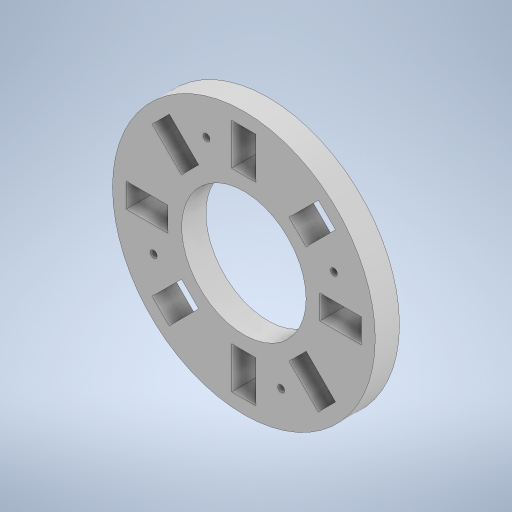
# Autodesk Inventor part: Spodnji obroc
Saved by Autodesk Inventor 2023 (Build 270158000, 158)
## iProperties
Created: 2022-12-16
Part Number: Spodnji obroc
Material: Generic
Document SubType Name: Modeling
Designer: David Zindović
Density: 1 g/cm^3
Appearance: Default
Author: David Zindović
Autodesk Inventor part; units mm, degrees
ref_plane "YZ Plane" through (0, 0, 0) normal (1, 0, 0) x (0, 1, 0)
ref_plane "XZ Plane" through (0, 0, 0) normal (0, 1, 0) x (-1, 0, 0)
ref_plane "XY Plane" through (0, 0, 0) normal (0, 0, 1) x (1, 0, 0)
sketch "Sketch1" plane through (0, 0, 0) normal (0, 0, 1) x (1, 0, 0)
  circle A0 centre (0, 0) radius 11
  circle A1 centre (0, 0) radius 17
  line L0 (11, 1.75) -> (17, 1.75)
  line L1 (17, 1.75) -> (17, -1.75)
  line L2 (17, -1.75) -> (11, -1.75)
  line L3 (11, -1.75) -> (11, 1.75)
  line L4 (13.2583, 10.7834) -> (9.0156, 6.5407)
  line L5 (9.0156, 6.5407) -> (6.5407, 9.0156)
  line L6 (6.5407, 9.0156) -> (10.7834, 13.2583)
  line L7 (10.7834, 13.2583) -> (13.2583, 10.7834)
  line L8 (1.75, 17) -> (1.75, 11)
  line L9 (1.75, 11) -> (-1.75, 11)
  line L10 (-1.75, 11) -> (-1.75, 17)
  line L11 (-1.75, 17) -> (1.75, 17)
  line L12 (-10.7834, 13.2583) -> (-6.5407, 9.0156)
  line L13 (-6.5407, 9.0156) -> (-9.0156, 6.5407)
  line L14 (-9.0156, 6.5407) -> (-13.2583, 10.7834)
  line L15 (-13.2583, 10.7834) -> (-10.7834, 13.2583)
  line L16 (-17, 1.75) -> (-11, 1.75)
  line L17 (-11, 1.75) -> (-11, -1.75)
  line L18 (-11, -1.75) -> (-17, -1.75)
  line L19 (-17, -1.75) -> (-17, 1.75)
  line L20 (-13.2583, -10.7834) -> (-9.0156, -6.5407)
  line L21 (-9.0156, -6.5407) -> (-6.5407, -9.0156)
  line L22 (-6.5407, -9.0156) -> (-10.7834, -13.2583)
  line L23 (-10.7834, -13.2583) -> (-13.2583, -10.7834)
  line L24 (-1.75, -17) -> (-1.75, -11)
  line L25 (-1.75, -11) -> (1.75, -11)
  line L26 (1.75, -11) -> (1.75, -17)
  line L27 (1.75, -17) -> (-1.75, -17)
  line L28 (10.7834, -13.2583) -> (6.5407, -9.0156)
  line L29 (6.5407, -9.0156) -> (9.0156, -6.5407)
  line L30 (9.0156, -6.5407) -> (13.2583, -10.7834)
  line L31 (13.2583, -10.7834) -> (10.7834, -13.2583)
  circle A2 centre (0, 0) radius 9
  circle A3 centre (0, 0) radius 19
  line L32 (-13.035, -5.3993) -> (-5.3993, 13.035)
  line L33 (-5.3993, 13.035) -> (13.035, 5.3993)
  line L34 (13.035, 5.3993) -> (5.3993, -13.035)
  line L35 (5.3993, -13.035) -> (-13.035, -5.3993)
  line L36 (0, 0) -> (-5.3993, 13.035)
  line L37 (0, 0) -> (14.109, 0) construction
  line L38 (0, 0) -> (16.0476, 6.6471)
  line L39 (0, 0) -> (17.3698, 0) construction
  circle A4 centre (-5.3993, 13.035) radius 0.5
  circle A5 centre (13.035, 5.3993) radius 0.5
  circle A6 centre (5.3993, -13.035) radius 0.5
  circle A7 centre (-13.035, -5.3993) radius 0.5
  point P0 (11, 0)
  point P1 (7.7782, 7.7782)
  point P2 (0, 11)
  point P3 (-7.7782, 7.7782)
  point P4 (-11, 0)
  point P5 (-7.7782, -7.7782)
  point P6 (0, -11)
  point P7 (7.7782, -7.7782)
  dimension "d0" = 22
  dimension "d1" = 6
  dimension "d2" = 3.5
  dimension "d3" = 6
  dimension "d6" = 360
  dimension "d8" = 2
  dimension "d9" = 2
  dimension "d23" = 112.5
  dimension "d24" = 22.5
  dimension "d25" = 1
  dimension "d26" = 1
  dimension "d27" = 1
  dimension "d28" = 1
  dimension "d29" = 14.109
  dimension "d30" = 19.9531
  dimension "d31" = 19.9531
  constraints: 81 end point, 8 centre point, 4 parallel, 3 coincident, 3 horizontal, 2 equal length, 2 perpendicular, 1 horizontal alignment, 1 midpoint, 1 point on line, 73 other
  measures "d0" diameter of A0
  measures "d1" radial gap between concentric circles of A0 A1
  measures "d2" distance of L2.end L0.start
  measures "d3" distance of L0.start L0.end
  measures "d8" radial gap between concentric circles of A0 A2
  measures "d9" radial gap between concentric circles of A1 A3
  measures "d23" angle of L37 L36
  measures "d24" angle of L39 L38
  measures "d25" diameter of A4
  measures "d26" diameter of A5
  measures "d27" diameter of A6
  measures "d28" diameter of A7
  measures "d29" distance of L36.start L32.end
  measures "d30" distance of L32.end L33.end
  measures "d31" distance of L33.end L34.end
extrude "Extrusion1" add sketch "Sketch1" along normal mid plane 3.5 contours A0 L34 | L3 L2 A1 L30 L29 A0 | A0 L34 L3 | L34 A0 L35 L32 L36 A2 L38 | A0 L38 A5 L34 L0 L3 | L29 L34 A0 | L38 A2 L36 A0 L33 | A0 L33 L5 L4 A5 L38 | L34 L29 L28 A6 L35 L26 L25 A0 | L34 A5 L38 A1 L0 | L33 A0 | A0 L5 L33 | L35 L25 A0 | A0 L35 | L28 A1 L26 L35 A6 L34 | A0 L9 L8 A1 L6 L5 | L33 L9 A0 | A0 L36 A4 L33 L10 L9 | L33 L4 A1 L38 A5 | L25 L24 A1 L22 L21 A0 | L35 L21 L20 A7 L32 L18 L17 A0 | A0 L21 L35 | A0 L32 L13 L12 A4 L36 | L32 L17 A0 | A0 L32 | A0 L13 L32 | L33 A4 L32 L12 A1 L10 | L17 L16 A1 L14 L13 A0 | L20 A1 L18 L32 A7 L35 | A3
equation "\"d25\" = d28"
equation "\"d26\" = d28"
equation "\"d27\" = d28"
body "Solid1"
